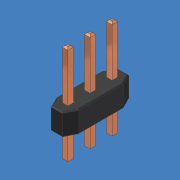
# Autodesk Inventor part: 3 Pin Connector
Saved by Autodesk Inventor 2014 SP1 (Build 180222100, 222)
## iProperties
Shininess: 64.0
Length Units: 11272
Angle Units: 11279
Time Units: 11290
Mass Units: 11286
Length Display Precision: 3
Angle Display Precision: 2
Compacted: True
Part Number: 3 Pin Connector
Document SubType Name: Modeling
Created: 2005-12-26
Designer: Owner
Material: ABS Plastic
Density: 1 g/cm^3
Appearance: Rubber - Black - Version 1.1
Density: 0.0
Volumn: 0.0
Area: 0.0
PropertySet Name: Model Information
Control State: 0
Master: False
Checked Out: False
Author: Owner
Autodesk Inventor part; units mm, degrees
ref_plane "YZ Plane" through (0, 0, 0) normal (1, 0, 0) x (0, 1, 0)
ref_plane "XZ Plane" through (0, 0, 0) normal (0, 1, 0) x (-1, 0, 0)
sketch "Sketch1" plane through (0, 0, 0) normal (0, 0, 1) x (1, 0, 0)
  line L0 (0, 0) -> (2.54, 0)
  line L1 (2.54, 0) -> (2.54, 7.62)
  line L2 (2.54, 7.62) -> (0, 7.62)
  line L3 (0, 7.62) -> (0, 0)
  line L4 (0.9525, 4.1275) -> (1.5875, 4.1275)
  line L5 (1.5875, 4.1275) -> (1.5875, 3.4925)
  line L6 (1.5875, 3.4925) -> (0.9525, 3.4925)
  line L7 (0.9525, 3.4925) -> (0.9525, 4.1275)
  line L8 (0.9525, 1.5875) -> (1.5875, 1.5875)
  line L9 (1.5875, 1.5875) -> (1.5875, 0.9525)
  line L10 (1.5875, 0.9525) -> (0.9525, 0.9525)
  line L11 (0.9525, 0.9525) -> (0.9525, 1.5875)
  line L12 (0.9525, 3.81) -> (0, 3.81)
  line L13 (1.5875, 1.27) -> (2.54, 1.27)
  line L14 (0.9525, 6.0325) -> (1.5875, 6.0325)
  line L15 (1.5875, 6.0325) -> (1.5875, 6.6675)
  line L16 (1.5875, 6.6675) -> (0.9525, 6.6675)
  line L17 (0.9525, 6.6675) -> (0.9525, 6.0325)
  dimension "d3" = 2.54
  dimension "d4" = 7.62
  dimension "d5" = 0.635
  dimension "d6" = 2.54
  dimension "d7" = 0.9525
  dimension "d25" = 2.54
  constraints: 36 end point, 8 parallel, 6 equal length, 6 perpendicular, 4 horizontal, 3 midpoint, 2 collinear, 1 point on line, 1 other
  measures "d3" distance of L0.start L0.end
  measures "d4" distance of L2.end L0.start
  measures "d5" distance of L4.end L5.end
  measures "d6" distance between parallel lines of L10 L6
  measures "d7" distance between parallel lines of L0 L10
  measures "d25" distance between parallel lines of L16 L4
extrude "Extrusion1" add sketch "Sketch1" along normal blind 2.54
chamfer "Chamfer1" distance 1.27 distance2 0.635 1 edges at (2.54, 7.62, 1.27) measured on face at (2.54, 3.3867, 0.8467)
chamfer "Chamfer2" distance 1.27 distance2 0.635 1 edges at (0, 7.62, 1.27) measured on face at (0, 6.35, 0.8467)
chamfer "Chamfer3" distance 1.27 distance2 0.635 1 edges at (0, 0, 1.27) measured on face at (0, 2.54, 0.8467)
chamfer "Chamfer4" distance 1.27 distance2 0.635 1 edges at (2.54, 0, 1.27) measured on face at (2.54, 0.4233, 0.8467)
ref_plane "Work Plane1" through (0, 0, -3.175) normal (0, 0, -1) x (-1, 0, 0)
sketch "Sketch2" plane through (0, 0, -3.175) normal (0, 0, -1) x (-1, 0, 0)
  line L0 (-1.5875, 4.1275) -> (-0.9525, 4.1275) projected
  line L1 (-1.5875, 3.4925) -> (-1.5875, 4.1275) projected
  line L2 (-0.9525, 4.1275) -> (-0.9525, 3.4925) projected
  line L3 (-0.9525, 3.4925) -> (-1.5875, 3.4925) projected
  line L4 (-1.5875, 1.5875) -> (-0.9525, 1.5875) projected
  line L5 (-0.9525, 1.5875) -> (-0.9525, 0.9525) projected
  line L6 (-0.9525, 0.9525) -> (-1.5875, 0.9525) projected
  line L7 (-1.5875, 0.9525) -> (-1.5875, 1.5875) projected
  line L8 (-0.9525, 6.6675) -> (-0.9525, 6.0325) projected
  line L9 (-0.9525, 6.0325) -> (-1.5875, 6.0325) projected
  line L10 (-1.5875, 6.0325) -> (-1.5875, 6.6675) projected
  line L11 (-1.5875, 6.6675) -> (-0.9525, 6.6675) projected
extrude "Extrusion2" add sketch "Sketch2" against normal blind 11.43
chamfer "Chamfer5" distance 0.1778 angle 45 24 edges at (1.5875, 1.27, 8.255) (1.27, 0.9525, 8.255) (0.9525, 1.27, 8.255) (1.27, 1.5875, 8.255) (1.27, 3.4925, 8.255) (1.5875, 3.81, 8.255) (1.27, 4.1275, 8.255) (0.9525, 3.81, 8.255) (1.5875, 1.27, -3.175) (1.27, 0.9525, -3.175) (0.9525, 1.27, -3.175) (1.27, 1.5875, -3.175) (1.27, 3.4925, -3.175) (0.9525, 3.81, -3.175) (1.27, 4.1275, -3.175) (1.5875, 3.81, -3.175) (1.27, 6.0325, 8.255) (0.9525, 6.35, 8.255) (1.27, 6.6675, 8.255) (1.5875, 6.35, 8.255) (1.5875, 6.35, -3.175) (1.27, 6.0325, -3.175) (0.9525, 6.35, -3.175) (1.27, 6.6675, -3.175)
chamfer "Chamfer6" distance 0.127 angle 45 16 edges at (2.54, 3.8099, 2.54) (2.2226, 0.635, 2.54) (1.27, 0, 2.54) (0.3175, 0.635, 2.54) (0, 3.81, 2.54) (0.3175, 6.985, 2.54) (1.27, 7.62, 2.54) (2.2225, 6.985, 2.54) (2.2225, 6.985, 0) (2.54, 3.8099, 0) (2.2226, 0.635, 0) (1.27, 0, 0) (0.3175, 0.635, 0) (0, 3.81, 0) (0.3175, 6.985, 0) (1.27, 7.62, 0)
body "Solid1"
